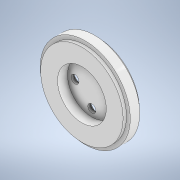
# Autodesk Inventor part: Колесо D40 под планшайбу
Saved by Autodesk Inventor 2020 (Build 240168000, 168)
## iProperties
Created: 2021-03-15
Part Number: Колесо D40 под планшайбу
Material: Типовые
Document SubType Name: Modeling
Designer: Антон
Density: 1 g/cm^3
Appearance: Белый
Author: Антон
Autodesk Inventor part; units mm, degrees
ref_plane "YZ Plane" through (0, 0, 0) normal (1, 0, 0) x (0, 1, 0)
ref_plane "XZ Plane" through (0, 0, 0) normal (0, 1, 0) x (-1, 0, 0)
ref_plane "XY Plane" through (0, 0, 0) normal (0, 0, 1) x (1, 0, 0)
sketch "Эскиз6" plane through (0, 0, 0) normal (0, 0, 1) x (1, 0, 0)
  circle A0 centre (0, 0) radius 18
  dimension "d27" = 36
  constraints: 1 centre point, 1 coincident
  measures "d27" diameter of A0
extrude "Выдавливание5" add sketch "Эскиз6" along normal blind 1.9
sketch "Эскиз7" plane through (0, 0, 1.9) normal (0, 0, 1) x (1, 0, 0)
  circle A0 centre (0, 0) radius 16.5
  dimension "d30" = 33
  constraints: 1 centre point, 1 coincident
  measures "d30" diameter of A0
extrude "Выдавливание6" add sketch "Эскиз7" along normal blind 1.35
mirror "Зеркальное отражение1" about plane through (0, 0, 0) normal (0, 0, -1)
sketch "Эскиз8" plane through (0, 0, 3.25) normal (0, 0, 1) x (1, 0, 0)
  circle A0 centre (0, 0) radius 9.75
  dimension "d33" = 19.5
  constraints: 1 centre point, 1 coincident
  measures "d33" diameter of A0
extrude "Выдавливание7" cut sketch "Эскиз8" against normal blind 4
sketch "Эскиз9" plane through (0, 0, -3.25) normal (0, 0, -1) x (-1, 0, 0)
  circle A0 centre (0, 0) radius 9.75 projected
  circle A1 centre (0, 0) radius 6.75 construction
  line L0 (0, -6.75) -> (0, 6.75) construction
  line L1 (-6.75, 0) -> (6.75, 0) construction
  dimension "d44" = 13.5
  constraints: 4 end point, 4 point on circle, 2 midpoint, 1 centre point, 1 coincident, 1 perpendicular, 1 vertical
  measures "d44" diameter of A1
hole "Отверстие2" at (0, 6.75, -3.25) at (6.75, 0, -3.25) at (-6.75, 0, -3.25) at (0, -6.75, -3.25) direction (0, 0, 1) diameter 3.2 end through all countersink diameter 6 countersink angle 90
